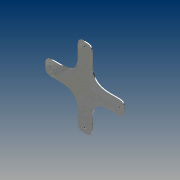
# Autodesk Inventor part: TopPlate
Saved by Autodesk Inventor 2011 SP1 (Build 150282100, 282)
## iProperties
Created: 2011-08-02
Part Number: TopPlate
Document SubType Name: Modeling
Designer: Nathan
Density: 1 g/cm^3
Author: Nathan
Autodesk Inventor part; units mm, degrees
ref_plane "YZ Plane" through (0, 0, 0) normal (1, 0, 0) x (0, 1, 0)
ref_plane "XZ Plane" through (0, 0, 0) normal (0, 1, 0) x (-1, 0, 0)
ref_plane "XY Plane" through (0, 0, 0) normal (0, 0, 1) x (1, 0, 0)
sketch "Sketch1" plane through (0, 0, 0) normal (0, 0, 1) x (1, 0, 0)
  spline S0 degree 5 poles (-66.04, 0) (-66.0342, -4.4696) (-65.2933, -11.8912) (-62.4015, -17.1256) (7.5159, 5.1628) (-23.6747, -81.3478) (0.2378, -55.6237) (23.6629, -81.762) (-6.9807, 7.0066) (81.862, -23.5409) (55.7411, -0.083) (81.8769, 23.8723) (-6.9695, -6.9946) (23.6659, 81.9149) (0.2329, 55.7231) (-23.6683, 81.5043) (7.4956, -5.219) (-62.4878, 17.435) (-65.3216, 11.9719) (-66.0458, 4.4778) (-66.04, 0) knots 0 0 0 0 0 0 0.074888 0.124865 0.182988 0.249885 0.316783 0.374906 0.433023 0.499862 0.566701 0.624819 0.682988 0.749885 0.816783 0.874952 0.924975 1 1 1 1 1 1
  line L0 (0, -6.1276) -> (0, 6.2502)
  line L1 (-5.7299, 0.0613) -> (8.1185, 0.0613)
  line L2 (0, 0) -> (10.1713, 10.1713)
  line L3 (0, 0) -> (14.3844, 0) construction
  point P0 (-18.941, -18.8184)
  point P1 (-10.1713, -63.1849)
  point P2 (0, -65.9787)
  point P3 (10.1713, -63.1849)
  point P4 (18.941, -18.8184)
  point P5 (63.3074, -10.0487)
  point P6 (66.04, 0)
  point P7 (63.3074, 10.1713)
  point P8 (18.941, 18.941)
  point P9 (10.1713, 63.3074)
  point P10 (0, 66.1013)
  point P11 (-10.1713, 63.3074)
  point P12 (-18.941, 18.941)
  point P13 (-63.3074, 10.1713)
  point P14 (0, 58.4813)
  point P15 (58.4813, 0)
  point P16 (0, -58.3587)
  point P17 (-58.4813, 0)
  dimension "d0" = 132.08
  dimension "d1" = 132.08
  dimension "d2" = 45
  dimension "d14" = 58.42
  constraints: 18 symmetric about line, 8 end point, 2 horizontal, 2 vertical, 1 equal length, 1 perpendicular, 1 point on line, 16 other
  measures "d0" distance of point (-66.04, 0) point (66.04, 0)
  measures "d1" distance of point (0, -65.979) point (0, 66.101)
  measures "d2" angle of L3 L2
  measures "d14" distance from line of L1 point (0, 58.481)
extrude "Extrusion1" add sketch "Sketch1" against normal blind 1.5875 contours S0 | L0 L1 L2
hole "Hole1" at (0, 58.4813, 0) at (58.4813, 0, 0) at (0, -58.3587, 0) at (-58.4813, 0, 0) direction (0, 0, -1) diameter 3.302 end through all thread size "8-32 UNC" class "2B" standard "ANSI Unified Screw Threads"
equation "\"d1\" = d0"
body "Solid1"
